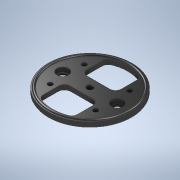
# Autodesk Inventor part: CarriageCap
Saved by Autodesk Inventor 2020 (Build 240168000, 168)
## iProperties
Created: 2019-06-07
Part Number: CarriageCap
Material: ABS Plastic
Document SubType Name: Modeling
Designer: Connor
Density: 1.06 g/cm^3
Appearance: Glossy - Black
Author: Connor
Autodesk Inventor part; units mm, degrees
ref_plane "YZ Plane" through (0, 0, 0) normal (1, 0, 0) x (0, 1, 0)
ref_plane "XZ Plane" through (0, 0, 0) normal (0, 1, 0) x (-1, 0, 0)
ref_plane "XY Plane" through (0, 0, 0) normal (0, 0, 1) x (1, 0, 0)
sketch "Sketch1" plane through (0, 0, 0) normal (0, 0, 1) x (1, 0, 0)
  line L0 (0, 0) -> (46.99, 0)
  line L1 (46.99, 0) -> (46.99, 6.35)
  line L2 (46.99, 6.35) -> (0, 6.35)
  line L3 (0, 6.35) -> (0, 0)
  circle A0 centre (44.45, 6.35) radius 1.397
  point P0 (45.847, 6.35)
  point P1 (43.053, 6.35)
  dimension "d0" = 46.99
  dimension "d1" = 6.35
  dimension "d2" = 44.45
  dimension "d3" = 2.794
  constraints: 8 end point, 2 parallel, 1 centre point, 1 horizontal, 1 perpendicular, 1 point on line
  measures "d0" distance of L2.end L1.end
  measures "d1" distance of L0.end L1.end
  measures "d2" distance from line of L3 A0.centre
  measures "d3" diameter of A0
revolve "Revolution1" add sketch "Sketch1" angle 360 about axis through (0, 6.35, 0) along (0, -1, 0)
sketch "Sketch4" plane through (0, 6.35, 0) normal (0, 1, 0) x (1, 0, 0)
  circle A0 centre (0, 0) radius 30.48 construction
  line L0 (-30.48, 0) -> (30.48, 0) construction
  dimension "d24" = 60.96
  constraints: 2 end point, 2 point on circle, 1 centre point, 1 coincident, 1 horizontal, 1 midpoint
  measures "d24" diameter of A0
hole "Hole2" at (-30.48, 6.35, 0) at (30.48, 6.35, 0) direction (0, -1, 0) diameter 8.89 end through all counterbore diameter 12.954 counterbore depth 4.7752
sketch "Sketch5" plane through (0, 6.35, 0) normal (0, 1, 0) x (1, 0, 0)
  arc A0 (-2.1767, 2.3114) -> (2.1767, 2.3114) centre (0, 0) ccw
  line L0 (-2.1767, 2.3114) -> (2.1767, 2.3114)
  line L1 (2.2753, 2.5654) -> (-2.2753, 2.5654)
  arc A1 (-2.2753, 2.5654) -> (2.2753, 2.5654) centre (0, 0) ccw
  arc A2 (2.2753, 2.5654) -> (-2.2753, 2.5654) centre (0, 0) ccw
  dimension "d32" = 6.35
  dimension "d33" = 5.4864
  dimension "d44" = 0.254
  constraints: 6 point on circle, 4 end point, 3 centre point, 2 coincident, 1 horizontal, 1 other
  measures "d32" diameter of A0
  measures "d44" radial gap between concentric circles of A0 A1
extrude "Extrusion2" cut sketch "Sketch5" against normal through all contours L0 A0 | A1 L1
sketch "Sketch6" plane through (0, 6.35, 0) normal (0, 1, 0) x (1, 0, 0)
  circle A0 centre (0, 0) radius 41.91
  line L0 (-19.05, 37.3302) -> (-19.05, -37.3302)
  line L1 (19.05, 37.3302) -> (19.05, -37.3302)
  line L2 (-40.8133, 9.525) -> (40.8133, 9.525)
  line L3 (40.8133, -9.525) -> (-40.8133, -9.525)
  point P0 (19.05, -9.525)
  point P1 (-19.05, -9.525)
  point P2 (-19.05, 9.525)
  point P3 (19.05, 9.525)
  dimension "d36" = 83.82
  dimension "d37" = 38.1
  dimension "d38" = 19.05
  constraints: 8 end point, 3 parallel, 2 vertical, 1 coincident, 1 horizontal, 10 other
  measures "d37" distance between parallel lines of L1 L0
  measures "d38" distance between parallel lines of L3 L2
extrude "Extrusion3" cut sketch "Sketch6" against normal blind 25.4 contours L1 L2 L0 A0 | A0 L0 L3 L1
fillet "Fillet1" radius 6.35 8 edges at (-19.05, 3.175, -37.3302) (-19.05, 3.175, 37.3302) (19.05, 3.175, -37.3302) (19.05, 3.175, 37.3302) (-19.05, 3.175, 9.525) (19.05, 3.175, 9.525) (-19.05, 3.175, -9.525) (19.05, 3.175, -9.525)
fillet "Fillet2" radius 1.5875 17 edges at (-46.99, 0, 0) (17.1901, 0, -11.3849) (17.9308, 0, -36.8149) (17.1901, 0, 11.3849) (17.9308, 0, 36.8149) (19.05, 0, -24.5449) (19.05, 0, 24.5449) (0, 0, -41.91) (0, 0, 41.91) (-17.9308, 0, -36.8149) (-17.9308, 0, 36.8149) (-19.05, 0, -24.5449) (-19.05, 0, 24.5449) (-17.1901, 0, -11.3849) (-17.1901, 0, 11.3849) (0, 0, -9.525) (0, 0, 9.525)
sketch "Sketch8" plane through (0, 0, 0) normal (0, -1, 0) x (1, 0, 0)
  line L0 (25.4, -19.05) -> (-25.4, -19.05) construction
  line L1 (-25.4, -19.05) -> (-25.4, 19.05) construction
  line L2 (-25.4, 19.05) -> (25.4, 19.05) construction
  line L3 (25.4, 19.05) -> (25.4, -19.05) construction
  line L4 (25.4, -19.05) -> (-25.4, 19.05) construction
  line L5 (25.4, 19.05) -> (-25.4, -19.05) construction
  point P0 (0, 0)
  point P1 (0, 0)
  dimension "d53" = 50.8
  dimension "d54" = 38.1
  constraints: 12 end point, 2 parallel, 1 coincident, 1 horizontal, 1 midpoint, 1 perpendicular
  measures "d53" distance of L0.start L0.end
  measures "d54" distance of L2.end L0.start
hole "Hole3" at (25.4, 0, -19.05) at (-25.4, 0, -19.05) at (-25.4, 0, 19.05) at (25.4, 0, 19.05) direction (0, 1, 0) diameter 5.207 depth 25.4
body "Solid1"
